# Autodesk Inventor part: Zahnriemen
Saved by Autodesk Inventor 2015 SP1 (Build 190203100, 203)
## iProperties
Created: 2015-03-05
Part Number: Zahnriemen
Material: Rubber
Document SubType Name: Modeling
Designer: Marc
Density: 1 g/cm^3
Appearance: Rubber - Black - Version 1.1
CustomPartVersion: 1
Author: Marc
Autodesk Inventor part; units mm, degrees
sketch "Skizzenpfad" plane through (0, 0, 0) normal (0, 0, 1) x (1, 0, 0)
  arc A0 (-6.0036, 3.9052) -> (0.7147, -7.1262) centre (0, 0) ccw
  arc A1 (33.5, 58.662) -> (27.4964, 55.4052) centre (33.5, 51.5) ccw
  arc A2 (514.2147, 44.3738) -> (513.5, 58.662) centre (513.5, 51.5) ccw
  line L0 (514.2147, 44.3738) -> (0.7147, -7.1262)
  line L1 (-6.0036, 3.9052) -> (27.4964, 55.4052)
  line L2 (33.5, 58.662) -> (513.5, 58.662)
  constraints: 6 end point, 6 point on circle, 3 centre point
ref_plane "Querschnittsebene" through (0.7147, -7.1262, 0) normal (0.995, 0.0998, 0) x (0, 0, 1)
ref_plane "Arbeitsebene2" through (0, 0, 0) normal (-1, 0, 0) x (0, 0, 1)
ref_plane "Arbeitsebene3" through (33.5, 51.5, 0) normal (-0.6226, -0.7826, 0) x (0, 0, 1)
ref_plane "Arbeitsebene4" through (513.5, 51.5, 0) normal (-0.8788, 0.4772, 0) x (0, 0, 1)
sketch "Querschnitt" plane through (0.7147, -7.1262, 0) normal (0.995, 0.0998, 0) x (0, 0, 1)
  line L0 (-3, 0.5) -> (3, 0.5)
  line L1 (3, 0.5) -> (3, -0.5)
  line L2 (3, -0.5) -> (-3, -0.5)
  line L3 (-3, -0.5) -> (-3, 0.5)
  line L4 (-3, 0) -> (3, 0) construction
  point P0 (0, 0)
  point P1 (0, 0)
  dimension "d0" = 6
  dimension "d4" = 0.5
  dimension "d5" = 0.5
  constraints: 10 end point, 3 midpoint, 2 parallel, 1 coincident, 1 horizontal, 1 perpendicular, 1 other
  measures "d0" distance between parallel lines of L1 L3
  measures "d4" distance between parallel lines of L2 L4
  measures "d5" distance between parallel lines of L4 L0
sweep "Riemen" add profiles "Querschnitt" path "Skizzenpfad"
equation "\"d0\" = da_B"
equation "\"d4\" = da_a"
equation "\"d5\" = da_a2"
equation "\"da_B\" = 6"
equation "\"da_pb\" = 5"
equation "\"da_L\" = 1102.51302"
equation "\"da_a\" = 0.5"
equation "\"da_S\" = 2.65"
equation "\"da_Beta\" = 20deg"
equation "\"da_Ht\" = 1.2"
equation "\"da_H\" = 2.2"
equation "\"da_a2\" = 0.5"
body "Solid1"
